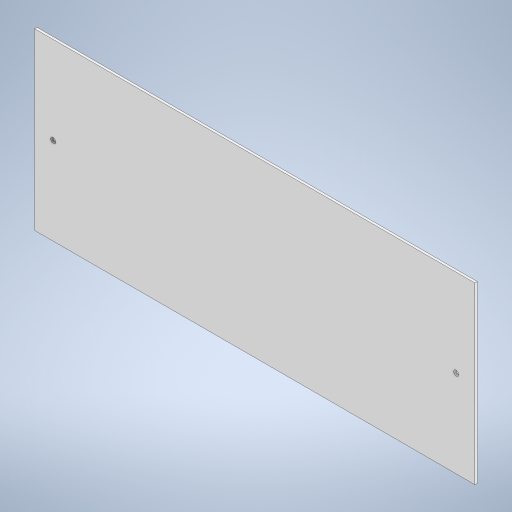
# Autodesk Inventor part: plate_top_01
Saved by Autodesk Inventor 2023 (Build 270158000, 158)
## iProperties
Created: 2023-08-22
Part Number: plate_top_01
Material: Polystyrene
Document SubType Name: Modeling
Designer: chriboehm
Density: 1.021 g/cm^3
Appearance: White
Author: chriboehm
Autodesk Inventor part; units mm, degrees
ref_plane "YZ Plane" through (0, 0, 0) normal (1, 0, 0) x (0, 1, 0)
ref_plane "XZ Plane" through (0, 0, 0) normal (0, 1, 0) x (-1, 0, 0)
ref_plane "XY Plane" through (0, 0, 0) normal (0, 0, 1) x (1, 0, 0)
sketch "Sketch1" plane through (0, 0, 0) normal (0, 0, 1) x (1, 0, 0)
  line L0 (0, 0) -> (542, 0)
  line L1 (542, 0) -> (542, 215)
  line L2 (542, 215) -> (0, 215)
  line L3 (0, 215) -> (0, 0)
  dimension "d0" = 542
  dimension "d1" = 215
  constraints: 8 end point, 2 parallel, 1 horizontal, 1 perpendicular
  measures "d0" distance of L1.end L2.end
  measures "d1" distance of L2.end L0.start
extrude "Extrusion1" add sketch "Sketch1" along normal blind 3
sketch "Sketch2" plane through (0, 0, 0) normal (0, 0, -1) x (-1, 0, 0)
  line L0 (0, 215) -> (0, 0) projected
  line L1 (0, 107.5) -> (-542, 107.5)
  line L2 (-542, 0) -> (-542, 215) projected
  point P0 (-23, 107.5)
  point P1 (-519, 107.5)
  dimension "d4" = 23
  dimension "d5" = 23
  constraints: 2 end point, 2 midpoint, 2 point on line, 1 perpendicular
  measures "d4" distance from line of L0 point (-23, 107.5)
  measures "d5" distance from line of L2 point (-519, 107.5)
hole "Hole1" at (23, 107.5, 0) at (519, 107.5, 0) direction (0, 0, 1) diameter 6.5 end through all
equation "\"d5\" = d4"
body "Solid1"
